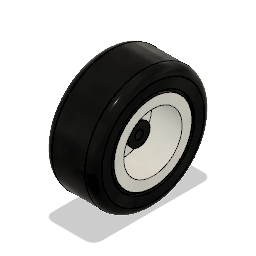
_k346 43x19x3mm wheel.aefafec7-2804-4509-a28a-ab8cc24bd11c (Autodesk Fusion 360 design; units mm, degrees)
Autodesk Fusion 360 part; units mm, degrees
note: some values were not read from the file. Chosen so that the rebuilt part matches the saved one: which face or edge a step refers to.
sketch "Sketch1" plane through (0, 0, 0) normal (0, 0, 1) x (1, 0, 0)
  line L0 (0, 0) -> (9, 0)
  line L1 (9, 12) -> (0, 12)
  line L2 (0, 12) -> (0, 0)
  line L3 (9, 12) -> (9, 0)
  dimension "d3" = 9
  dimension "d4" = 12
  dimension "d6" = 12
  measures "d3" distance of L0.start
  measures "d4" distance of L0.start
sketch "Sketch2" plane through (24, 0, 0) normal (1, 0, 0) x (0, 0, -1)
  line L0 (0, 0) -> (0, 12)
  line L1 (0, 12) -> (-10, 12)
  line L2 (-10, 12) -> (-10, 0)
  line L3 (-10, 0) -> (0, 0)
  line L4 (0, 2.6834) -> (0, 9.3166)
  line L5 (-10, 9.3166) -> (-10, 2.6834)
  arc A0 (-10, 2.6834) -> (0, 2.6834) centre (-5, 6) ccw
  arc A1 (0, 9.3166) -> (-10, 9.3166) centre (-5, 6) ccw
  circle A2 centre (-5, 6) radius 2.5
  circle A3 centre (-5, 6) radius 1.5
  circle A4 centre (-50, 25) radius 21.5
  circle A5 centre (-50, 25) radius 15
  circle A6 centre (-50, 25) radius 14
  circle A7 centre (-50, 25) radius 10.5
  circle A8 centre (-50, 25) radius 4
  circle A9 centre (-50, 25) radius 1.5
  dimension "d13" = 5
  dimension "d16" = 3
  dimension "d297" = 43
  dimension "d298" = 30
  dimension "d299" = 28
  dimension "d300" = 21
  dimension "d301" = 8
  dimension "d302" = 3
  measures "d13" diameter of A2
  measures "d16" diameter of A3
  measures "d297" diameter of A4
  measures "d298" diameter of A5
  measures "d299" diameter of A6
  measures "d300" diameter of A7
  measures "d301" diameter of A8
  measures "d302" diameter of A9
extrude "Extrude12" add sketch "Sketch2" along normal blind 14 contours A4 makes body 1
extrude "Extrude13" add sketch "Sketch2" against normal blind 4 contours A4 bodies 1
extrude "Extrude14" add sketch "Sketch2" along normal blind 14 separate body contours A6 makes body 2
extrude "Extrude15" add sketch "Sketch2" along normal blind 13 contours A5 bodies 1 2
extrude "Extrude17" add sketch "Sketch2" along normal blind 3 contours A7 bodies 1
extrude "Extrude18" add sketch "Sketch2" along normal blind 9 contours A8 bodies 1
fillet "Fillet1" radius 3 1 edges at (20, 25, 71.5) on bodies 1
fillet "Fillet2" radius 3 1 edges at (38, 17.2253, 70.045) on bodies 1
move_body "Move2" bodies 1 to x (1, 0, 0) y (0, 1, 0) z (0, 0, 1) at (-34, -19, -45)
